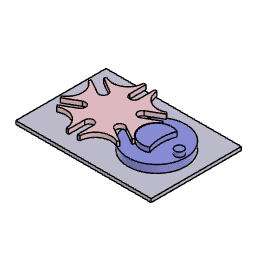
Geneva Mechanism (Autodesk Fusion 360 design; units mm, degrees)
Autodesk Fusion 360 part; units mm, degrees
sketch "Mechanism" plane through (0, 0, 0) normal (0, 0, 1) x (1, 0, 0)
  line L0 (14.9706, 13.2621) -> (27.7993, 20.6688)
  line L1 (18.9706, 6.3339) -> (31.7993, 13.7405)
  line L2 (-4, 19.5959) -> (-4, 34.4093)
  line L3 (4, 19.5959) -> (4, 34.4093)
  line L4 (-18.9706, 6.3339) -> (-31.7993, 13.7405)
  line L5 (-14.9706, 13.2621) -> (-27.7993, 20.6688)
  line L6 (-14.9706, -13.2621) -> (-27.7993, -20.6688)
  line L7 (-18.9706, -6.3339) -> (-31.7993, -13.7405)
  line L8 (4, -19.5959) -> (4, -34.4093)
  line L9 (-4, -19.5959) -> (-4, -34.4093)
  line L10 (18.9706, -6.3339) -> (31.7993, -13.7405)
  line L11 (14.9706, -13.2621) -> (27.7993, -20.6688)
  arc A0 (-26.5401, 22.2625) -> (-6.0099, 34.1157) centre (-20, 34.641) ccw
  arc A1 (6.0099, 34.1157) -> (26.5401, 22.2625) centre (20, 34.641) ccw
  arc A2 (-6.0099, -34.1157) -> (-26.5401, -22.2625) centre (-20, -34.641) ccw
  arc A3 (26.5401, -22.2625) -> (6.0099, -34.1157) centre (20, -34.641) ccw
  arc A4 (-32.55, -11.8532) -> (-32.55, 11.8532) centre (-40, 0) ccw
  arc A5 (-26.5401, 22.2625) -> (-27.8033, 20.6634) centre (0, 0) ccw
  arc A6 (-31.7967, 13.7467) -> (-32.55, 11.8532) centre (0, 0) ccw
  arc A7 (-32.55, -11.8532) -> (-31.7967, -13.7467) centre (0, 0) ccw
  arc A8 (-27.8033, -20.6634) -> (-26.5401, -22.2625) centre (0, 0) ccw
  arc A9 (-15.3205, -13.4641) -> (-19.3205, -6.5359) centre (-17.3205, -10) ccw
  arc A10 (-6.0099, -34.1157) -> (-3.9933, -34.4101) centre (0, 0) ccw
  arc A11 (3.9933, -34.4101) -> (6.0099, -34.1157) centre (0, 0) ccw
  arc A12 (4, -20) -> (-4, -20) centre (0, -20) ccw
  arc A13 (-19.3205, 6.5359) -> (-15.3205, 13.4641) centre (-17.3205, 10) ccw
  arc A14 (6.0099, 34.1157) -> (3.9933, 34.4101) centre (0, 0) ccw
  arc A15 (-3.9933, 34.4101) -> (-6.0099, 34.1157) centre (0, 0) ccw
  arc A16 (-4, 20) -> (4, 20) centre (0, 20) ccw
  arc A17 (26.5401, -22.2625) -> (27.8033, -20.6634) centre (0, 0) ccw
  arc A18 (19.3205, -6.5359) -> (15.3205, -13.4641) centre (17.3205, -10) ccw
  arc A19 (15.3205, 13.4641) -> (19.3205, 6.5359) centre (17.3205, 10) ccw
  arc A20 (27.7993, 20.6688) -> (26.5401, 22.2625) centre (0, 0) ccw
  arc A21 (31.7967, -13.7467) -> (32.55, -11.8532) centre (0, 0) ccw
  arc A22 (32.55, 11.8532) -> (31.7993, 13.7405) centre (0, 0) ccw
  circle A23 centre (60, 0) radius 4
  circle A24 centre (40, 0) radius 25.6061
  arc A25 (45.8442, 12.1694) -> (45.8442, -12.1694) centre (40, 0) ccw
  arc A26 (45.8442, 12.1694) -> (45.8442, -12.1694) centre (80, 0) ccw
  arc A27 (32.55, 11.8532) -> (32.55, -11.8532) centre (40, 0) ccw
  circle A28 centre (0, 0) radius 6
  circle A29 centre (0, 0) radius 3
  circle A30 centre (40, 0) radius 2.6
  circle A31 centre (40, 0) radius 6
  line L12 (75, 40) -> (-45, 40)
  line L13 (-45, 40) -> (-45, -40)
  line L14 (-45, -40) -> (75, -40)
  line L15 (75, -40) -> (75, 40)
  point P0 (14.3939, 0)
  dimension "d18" = 8
  constraint coincident A5.centre A6.centre
  constraint tangent L0 A19
  constraint tangent L1 A19
  constraint coincident A1.end A5
  constraint coincident A1.start A5
  constraint concentric A5 A14
  constraint coincident A2.start A5
  constraint coincident A3.end A5
  constraint coincident A3.start A5
  constraint concentric A5 A10
  constraint concentric A10 A17
  constraint coincident A8.start A5
  constraint coincident A7.end A5
  constraint coincident A4.start A5
  constraint concentric A5 A7
  constraint concentric A5 A6
  constraint concentric A7 A8
  constraint coincident A8 L6.end
  constraint coincident A7 L7.end
  constraint coincident L7 A9.end
  constraint coincident L6 A9.start
  constraint concentric A10 A11
  constraint coincident L9 A12.end
  constraint coincident L8 A12.start
  constraint coincident A10 L9.end
  constraint coincident A11 L8.end
  constraint coincident L5 A13.end
  constraint coincident L4 A13.start
  constraint coincident A6 L4.end
  constraint coincident A5 L5.end
  constraint concentric A14 A15
  constraint coincident L3 A16.end
  constraint coincident L2 A16.start
  constraint coincident A15 L2.end
  constraint coincident A14 L3.end
  constraint concentric A17 A21
  constraint coincident L11 A18.end
  constraint coincident L10 A18.start
  constraint coincident L10.end A21
  constraint coincident A17 L11.end
  constraint coincident L0 A19.start
  constraint coincident L1 A19.end
  constraint coincident L0.end A21
  constraint concentric A20 A21
  constraint coincident L1.end A21
  constraint concentric A21 A22
  constraint concentric A10 A28
  constraint concentric A8 A29
  constraint concentric A27 A30
  constraint concentric A30 A31
  constraint horizontal L12
  constraint perpendicular L12 L13
  constraint parallel L12 L14
  constraint parallel L13 L15
  constraint coincident A24 P0
  measures "d18" diameter of A23
extrude "Extrude1" add sketch "Mechanism" along normal blind 3 contours L0 L2 L3 L4 L5 L6 L7 L8 L9 L11 A0 A1 A2 A3 A4 A5 A6 A7 A8 A9 A10 A11 A12 A13 A14 A15 A16 A17 A18 A19 A20 A24 | L0 A19 A24 | L0 A20 A24 | L0 L1 L10 L11 A17 A18 A19 A20 A21 A22 A24 A27 | L1 L10 A18 A19 A21 A22 A24 A27 | L11 A18 A24 | L11 A17 A24 | A23 | A25 A26 A31 | A26 A31 | A26 A31 | A28 | A29 | A30 | L12 L13 L14 L15 makes body 1 in component "Base"
extrude "Extrude2" add sketch "Mechanism" along normal blind 8 contours A29 | A30 bodies 1 in component "Base"
extrude "Extrude1'" add sketch "Mechanism" along normal blind 11 and the other way blind -3 separate body contours A28 makes body 2 in component "Driven Wheel"
extrude "Extrude2'" add 1 faces at (-0.2426, 0.1169, 8) along direction (0, 0, 1) blind 3 on bodies 1 bodies 2 in component "Driven Wheel"
extrude "Extrude3" add sketch "Mechanism" along normal blind 14 and the other way blind -10 contours L0 L2 L3 L4 L5 L6 L7 L8 L9 L11 A0 A1 A2 A3 A4 A5 A6 A7 A8 A9 A10 A11 A12 A13 A14 A15 A16 A17 A18 A19 A20 A24 | L0 A20 A24 | L1 L10 A18 A19 A21 A22 A24 A27 | L11 A17 A24 bodies 2 in component "Driven Wheel"
extrude "Extrude4" add 1 faces at (-1.0665, 0.3664, 11) along direction (0, 0, 1) blind 3 on bodies 2 bodies 2 in component "Driven Wheel"
extrude "Extrude1''" add sketch "Mechanism" along normal blind 10 and the other way blind -3 separate body contours A26 A31 | A26 A31 makes body 3 in component "Rotating wheel"
extrude "Extrude2''" add sketch "Mechanism" along normal blind 10 and the other way blind -3 contours L0 A20 A24 | L0 L1 L10 L11 A17 A18 A19 A20 A21 A22 A24 A27 | L1 L10 A18 A19 A21 A22 A24 A27 | L11 A17 A24 | A23 | A25 A26 A31 bodies 3 in component "Rotating wheel"
extrude "Extrude3'" add 1 faces at (39.4386, 0.7699, 8) along direction (0, 0, 1) blind 2 on bodies 1 bodies 3 in component "Rotating wheel"
extrude "Extrude4'" add sketch "Mechanism" along normal blind 14 and the other way blind -10 contours A23 | A25 A26 A31 | A26 A31 | A30 picked at (43.2312, -2.5718) bodies 3 in component "Rotating wheel"
move_face "OffsetFaces1" offset -0.2 1 faces at (63.995, -0.1994, 12.6667) on bodies 3 in component "Rotating wheel"
move_face "OffsetFaces2" offset -0.2 1 faces at (55.0336, -9.9616, 10) on bodies 3 in component "Rotating wheel"
component "Base" placed x (1, 0, 0) y (0, 1, 0) z (0, 0, 1) at (0, 0, 0)
component "Driven Wheel" placed x (0.500168, -0.865928, 0) y (0.865928, 0.500168, 0) z (0, 0, 1) at (0, 0, 0)
component "Rotating wheel" placed x (1, 0, 0) y (0, 1, 0) z (0, 0, 1) at (0, 0, 0)
named bodies: "Base", "Driven Wheel", "Rotating Wheel"
